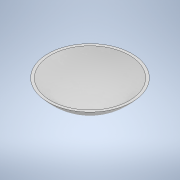
# Autodesk Inventor part: Main Mirror
Saved by Autodesk Inventor 2022 (Build 260153000, 153)
## iProperties
Created: 2023-08-20
Part Number: Main Mirror
Material: Generic
Document SubType Name: Modeling
Designer: fouad
Density: 1 g/cm^3
Appearance: Default
Author: fouad
Autodesk Inventor part; units mm, degrees
ref_plane "YZ Plane" through (0, 0, 0) normal (1, 0, 0) x (0, 1, 0)
ref_plane "XZ Plane" through (0, 0, 0) normal (0, 1, 0) x (-1, 0, 0)
ref_plane "XY Plane" through (0, 0, 0) normal (0, 0, 1) x (1, 0, 0)
sketch "Sketch2" plane through (0, 0, 0) normal (0, 0, 1) x (1, 0, 0)
  circle A0 centre (0, 0) radius 25
  circle A1 centre (0, 0) radius 24
  line L0 (-28.1544, -15) -> (30.7149, -15)
  line L1 (0, -25) -> (0, -24)
  point P0 (20, -15)
  point P1 (18.735, -15)
  dimension "d3" = 50
  dimension "d4" = 48
  dimension "d6" = 10
  constraints: 4 end point, 2 coincident, 1 horizontal, 1 perpendicular, 6 other
  measures "d6" distance from line of L0 L1.start
revolve "Revolution1" add sketch "Sketch2" angle 360 about axis through (0, -25, 0) along (0, 1, 0) picked at (16.5634, -17.6598) contours A0 L1 A1 L0
body "Solid2"
